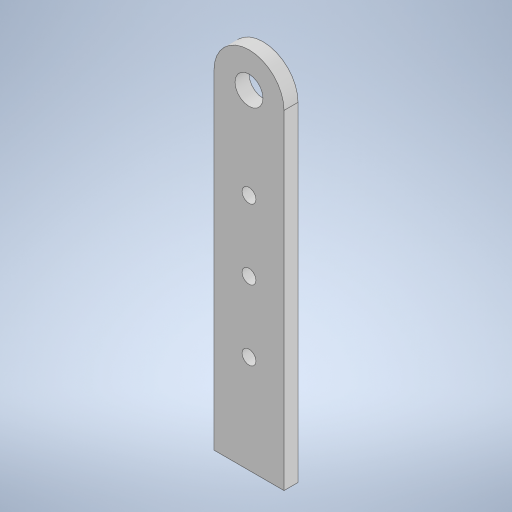
# Autodesk Inventor part: cutter_board
Saved by Autodesk Inventor 2024 (Build 280153000, 153)
## iProperties
Created: 2025-03-05
Part Number: cutter_board
Material: 一般
Document SubType Name: Modeling
Designer: 1412z
Density: 1 g/cm^3
Appearance: 既定
Author: 1412z
Autodesk Inventor part; units mm, degrees
ref_plane "YZ Plane" through (0, 0, 0) normal (1, 0, 0) x (0, 1, 0)
ref_plane "XZ Plane" through (0, 0, 0) normal (0, 1, 0) x (-1, 0, 0)
ref_plane "XY Plane" through (0, 0, 0) normal (0, 0, 1) x (1, 0, 0)
sketch "スケッチ1" plane through (0, 0, 0) normal (0, 0, 1) x (1, 0, 0)
  circle A0 centre (0, 0) radius 5
  circle A1 centre (0, 0) radius 2
  line L0 (0, -2) -> (0, -47)
  line L1 (5, 0) -> (5, -47)
  line L2 (5, -47) -> (-5, -47)
  line L3 (-5, -47) -> (-5, 0)
  circle A2 centre (0, -23) radius 1
  circle A3 centre (0, -13) radius 1
  circle A4 centre (0, -33) radius 1
  dimension "d1" = 4
  dimension "d0" = 10
  dimension "d2" = 45
  dimension "d3" = 2
  dimension "d4" = 2
  dimension "d5" = 2
  constraints: 8 end point, 4 centre point, 3 point on line, 2 coincident, 2 point on circle, 2 tangent, 2 vertical, 1 perpendicular, 1 vertical alignment, 2 other
  measures "d0" diameter of A0
  measures "d2" distance of L0.start L0.end
  measures "d3" diameter of A2
  measures "d4" diameter of A3
  measures "d5" diameter of A4
extrude "押し出し1" add sketch "スケッチ1" along normal blind 2 contours A0 | L1 L2 L0 A4 A2 A3 A0 | A0 L0 A3 A2 A4 L2 L3
